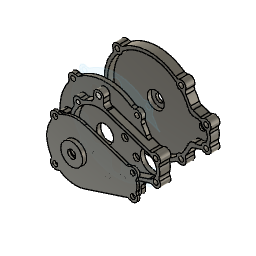
Gear Reduction Housing Assembly (v2~recovered) (Autodesk Fusion 360 design; units mm, degrees)
Autodesk Fusion 360 part; units mm, degrees
sketch "Layout Sketch" plane through (0, 0, 0) normal (0, 1, 0) x (1, 0, 0)
  circle A0 centre (0, 0) radius 48
  circle A1 centre (0, 0) radius 16
  circle A2 centre (58, 0) radius 10
  circle A3 centre (24.6564, -8.25) radius 10
  circle A4 centre (38.8667, 5.8237) radius 10
  line L0 (0, 0) -> (38.8667, 0) construction
  line L1 (38.8667, 0) -> (38.8667, 5.8237) construction
  line L2 (24.6564, -8.25) -> (24.6564, 0) construction
  circle A5 centre (38.8667, 5.8237) radius 14 construction
  circle A6 centre (24.6564, -8.25) radius 14 construction
  dimension "d12" = 96
  dimension "d13" = 32
  dimension "d14" = 20
  dimension "d15" = 20
  dimension "d16" = 20
  dimension "d55" = 4
  dimension "d56" = 8.25
  constraint coincident A0.centre A1.centre
  constraint concentric A0 A1
  constraint horizontal A0.centre A2.centre
  constraint tangent A0 A2
  constraint tangent A3 A4
  constraint tangent A1 A3
  constraint horizontal L0
  constraint coincident A4.centre L1.end
  constraint coincident A3.centre L2.start
  constraint coincident L0 L2.end
  constraint perpendicular L0 L2
  constraint perpendicular L0 L1
  constraint tangent A2 A4
  constraint concentric A4 A5
  constraint concentric A3 A6
  constraint equal A5 A6
  measures "d12" diameter of A0
  measures "d13" diameter of A1
  measures "d14" diameter of A2
  measures "d15" diameter of A3
  measures "d16" diameter of A4
  measures "d55" distance of A4 A5
  measures "d56" distance of A3.centre L2.end
sketch "Housing Layout Sketch" plane through (0, 0, 0) normal (0, 1, 0) x (1, 0, 0)
  circle A0 centre (0, 0) radius 56
  circle A1 centre (0, 0) radius 48 construction
  circle A2 centre (58, 0) radius 10 construction
  circle A3 centre (58, 0) radius 18
  circle A4 centre (39.598, 39.598) radius 6
  line L0 (0, 0) -> (0, 56) construction
  line L1 (0, 0) -> (39.598, 39.598) construction
  line L2 (0, 0) -> (-56, 0) construction
  circle A5 centre (-39.598, 39.598) radius 6
  circle A6 centre (-39.598, -39.598) radius 6
  circle A7 centre (39.598, -39.598) radius 6
  circle A8 centre (70.7279, -12.7279) radius 6
  line L3 (58, 0) -> (70.7279, -12.7279) construction
  circle A9 centre (70.7279, 12.7279) radius 6
  circle A10 centre (39.598, 39.598) radius 4
  circle A11 centre (-39.598, 39.598) radius 4
  circle A12 centre (-39.598, -39.598) radius 4
  circle A13 centre (39.598, -39.598) radius 4
  circle A14 centre (70.7279, -12.7279) radius 4
  circle A15 centre (70.7279, 12.7279) radius 4
  circle A16 centre (0, 0) radius 16 construction
  circle A17 centre (24.6564, -8.25) radius 10 construction
  circle A18 centre (38.8667, 5.8237) radius 10 construction
  circle A19 centre (0, 0) radius 36
  line L4 (11.1724, -34.2225) -> (63.5862, -17.1112)
  line L5 (11.1724, 34.2225) -> (63.5862, 17.1112)
  circle A20 centre (24.6564, -8.25) radius 4
  circle A21 centre (38.8667, 5.8237) radius 4
  circle A22 centre (58, 0) radius 4
  circle A23 centre (0, 0) radius 52
  circle A24 centre (0, 0) radius 5
  circle A25 centre (58, 0) radius 14
  dimension "Gear_Clearance_Drive" = 8
  dimension "d18" = 8
  dimension "d19" = 12
  dimension "d20" = 45
  dimension "d21" = 45
  dimension "d22" = 8
  dimension "d23" = 20
  dimension "d24" = 8
  dimension "d25" = 104
  dimension "d27" = 10
  dimension "d57" = 4
  constraint coincident A0.centre A1.centre
  constraint coincident A0 A4.centre
  constraint coincident A0 L0.end
  constraint vertical L0
  constraint coincident A4.centre L1.end
  constraint coincident A0 L2.end
  constraint perpendicular L0 L2
  constraint symmetric A4 L0 A5
  constraint coincident A0 A6.centre
  constraint symmetric L2 A5 A6
  constraint coincident A0 A7.centre
  constraint symmetric L0 A6 A7
  constraint coincident A3 A8.centre
  constraint coincident A2.centre A3.centre
  constraint coincident A8.centre L3.end
  constraint equal A4 A8
  constraint symmetric L2 A8 A9
  constraint concentric A4 A10
  constraint concentric A5 A11
  constraint concentric A6 A12
  constraint concentric A7 A13
  constraint concentric A8 A14
  constraint concentric A9 A15
  constraint equal A14 A15
  constraint equal A13 A14
  constraint equal A12 A13
  constraint equal A11 A12
  constraint equal A10 A11
  constraint concentric A16 A19
  constraint coincident A19 L4.start
  constraint coincident A3 L4.end
  constraint coincident A19 L5.start
  constraint coincident A3 L5.end
  constraint tangent A19 L4
  constraint tangent A3 L4
  constraint tangent A19 L5
  constraint tangent A3 L5
  constraint concentric A17 A20
  constraint concentric A18 A21
  constraint equal A21 A22
  constraint equal A20 A21
  constraint concentric A16 A23
  constraint concentric A23 A24
  constraint concentric A22 A25
  measures "Gear_Clearance_Drive" distance of A0 A1
  measures "d19" diameter of A4
  measures "d20" angle of L0 L1
  measures "d21" angle of L0 L3
  measures "d22" diameter of A10
  measures "d23" distance of A16 A19
  measures "d24" diameter of A22
  measures "d25" diameter of A23
  measures "d27" diameter of A24
  measures "d57" distance of A2 A25
ref_plane "WorkPlane1" through (0, 11, 0) normal (0, 1, 0) x (0, 0, 1)
ref_plane "WorkPlane2" through (0, -5, 0) normal (0, 1, 0) x (0, 0, 1)
ref_plane "WorkPlane3" through (0, -13, 0) normal (0, 1, 0) x (0, 0, 1)
extrude "Extrude1" add sketch "Housing Layout Sketch" along normal up to surface (11 mm away) contours A0 A22 | A0 A22 | A0 A22 A23 A25 | A0 A8 A9 A22 A25 | A0 A3 A23 A25 | A0 A3 A9 A25 | A0 A3 A8 A25 | A0 A3 A23 A25 | A0 A3 L5 A23 | A0 A3 L5 | A9 A25 | A3 A9 A15 A25 | A3 A21 A23 A25 | A23 A25 | A0 A3 L4 | A0 A3 L4 A23 | A3 A8 A14 A25 | A8 A25 | A0 A4 L5 A23 | A3 A19 L5 A21 A23 | A3 A9 A15 | A3 A9 A15 A25 | A3 A8 A9 A25 | A3 A15 | A0 A7 L4 A23 | A3 A19 L4 A21 A23 | A3 A8 A14 A25 | A3 A8 A14 | A3 A14 | A0 A4 A10 A23 | A0 A4 A10 | A4 A5 A6 A7 A19 L4 L5 A23 | A3 A21 | A3 A19 A21 | A3 A15 | A0 A7 A13 | A0 A7 A13 A23 | A3 A14 | A0 A10 | A0 A10 | A4 A23 | A19 A21 | A19 A21 | A0 A13 | A0 A13 | A7 A23 | A0 A4 A10 A23 | A0 A4 A5 A23 | A0 A7 A13 A23 | A0 A6 A7 A23 | A0 A5 A11 A23 | A5 A23 | A0 A5 A11 | A0 A6 A12 | A0 A6 A12 A23 | A6 A23 | A0 A5 A11 A23 | A0 A11 | A0 A11 | A0 A5 A6 A23 | A0 A12 | A0 A12 | A0 A6 A12 A23 | A20 | A24 makes body 1
extrude "Extrude2" add 1 faces at (5.6052, 0, -26.2324) along direction (0, -1, 0) up to surface (5 mm away) separate body on bodies 1 makes body 2
extrude "Extrude3" add sketch "Housing Layout Sketch" against normal up to surface (8 mm away) from surface at -5 separate body contours A0 A22 | A0 A22 | A0 A22 A23 A25 | A0 A8 A9 A22 A25 | A0 A3 A23 A25 | A0 A3 A9 A25 | A0 A3 A8 A25 | A0 A3 A23 A25 | A0 A3 L5 A23 | A0 A3 L5 | A9 A25 | A3 A9 A15 A25 | A3 A21 A23 A25 | A23 A25 | A0 A3 L4 | A0 A3 L4 A23 | A3 A8 A14 A25 | A8 A25 | A3 A19 L5 A21 A23 | A3 A9 A15 | A3 A9 A15 A25 | A3 A8 A9 A25 | A3 A15 | A3 A19 L4 A21 A23 | A3 A8 A14 A25 | A3 A8 A14 | A3 A14 | A3 A21 | A3 A19 A21 | A3 A15 | A3 A14 | A19 A21 | A19 A21 | A20 | A24 makes body 3
extrude "Extrude4" add 1 faces at (-6.1142, -13, -2.1538) along direction (0, -1, 0) blind 3 separate body on bodies 3 makes body 4
combine "Combine1" operation add target body 2 tool bodies 3
sketch "Front Cover Cut" plane through (0, -13, 0) normal (0, -1, 0) x (1, 0, 0)
  arc A0 (65.8375, 16.2041) -> (63.5862, 17.1112) centre (58, 0) ccw
  line L0 (63.5862, 17.1112) -> (11.1724, 34.2225)
  arc A1 (11.1724, 34.2225) -> (11.1724, -34.2225) centre (0, 0) ccw
  line L1 (11.1724, -34.2225) -> (63.5862, -17.1112)
  arc A2 (63.5862, -17.1112) -> (65.8375, -16.2041) centre (58, 0) ccw
  arc A3 (65.8375, -16.2041) -> (74.2041, -7.8375) centre (70.7279, -12.7279) ccw
  arc A4 (74.2041, -7.8375) -> (74.2041, 7.8375) centre (58, 0) ccw
  arc A5 (74.2041, 7.8375) -> (65.8375, 16.2041) centre (70.7279, 12.7279) ccw
  line L2 (11.1724, 34.2225) -> (63.5862, 17.1112)
  circle A6 centre (0, 0) radius 36 construction
  circle A7 centre (58, 0) radius 18 construction
  line L3 (11.1724, -34.2225) -> (63.5862, -17.1112)
  arc A8 (11.1724, 34.2225) -> (11.1724, -34.2225) centre (0, 0) ccw
  arc A9 (63.5862, -17.1112) -> (63.5862, 17.1112) centre (58, 0) ccw
  arc A10 (62.3448, -13.3087) -> (62.3448, 13.3087) centre (58, 0) ccw
  line L4 (62.3448, 13.3087) -> (9.931, 30.42)
  arc A11 (9.931, 30.42) -> (9.931, -30.42) centre (0, 0) ccw
  line L5 (9.931, -30.42) -> (62.3448, -13.3087)
  dimension "d44" = -4
  constraint coincident A1.end L1.start
  constraint coincident L0.end A1.start
  constraint tangent L0 A8
  constraint coincident A0.end L0.start
  constraint coincident L1.end A2.start
  constraint tangent L3 A9
extrude "Extrude5" cut sketch "Front Cover Cut" against normal up to surface (8 mm away) contours A10 L4 A11 L5 bodies 2
sketch "Main Bearing OD" plane through (0, 0, 0) normal (0, 1, 0) x (1, 0, 0)
  circle A0 centre (0, 0) radius 10.5
  dimension "d47" = 21
  constraint coincident A0.centre origin
  measures "d47" diameter of A0
extrude "Extrude6" cut sketch "Main Bearing OD" along normal through all and the other way through all bodies 1 2 4
sketch "Cover Bearing" plane through (0, 0, 0) normal (1, 0, 0) x (0, 1, 0)
  line L0 (-13, -10.5) -> (-16, -10.5)
  line L1 (-16, 10.5) -> (-13, 10.5)
  line L2 (-16, 10.5) -> (-18, 10.5)
  line L3 (-18, 10.5) -> (-18, 5)
  line L4 (-18, 5) -> (-21, 5)
  line L5 (-21, 5) -> (-21, 13.5)
  line L6 (-21, 13.5) -> (-16, 13.5)
  line L7 (-16, 13.5) -> (-16, 10.5)
  line L8 (0, 0) -> (-21.9581, 0) construction
  line L9 (11, -10.5) -> (0, -10.5)
  line L10 (0, 10.5) -> (11, 10.5)
  line L11 (11, 10.5) -> (13, 10.5)
  line L12 (13, 10.5) -> (13, 5)
  line L13 (13, 5) -> (16, 5)
  line L14 (16, 5) -> (16, 13.5)
  line L15 (16, 13.5) -> (11, 13.5)
  line L16 (11, 13.5) -> (11, 10.5)
  dimension "d49" = 5
  dimension "d50" = 3
  dimension "d51" = 3
  dimension "d52" = 10
  constraint coincident L1.start L2.start
  constraint parallel L1 L2
  constraint perpendicular L2 L3
  constraint perpendicular L3 L4
  constraint perpendicular L2 L5
  constraint perpendicular L5 L6
  constraint perpendicular L2 L7
  constraint coincident L8.start origin
  constraint parallel L6 L8
  constraint coincident L10.end L11.start
  constraint parallel L10 L11
  constraint perpendicular L11 L12
  constraint perpendicular L12 L13
  constraint perpendicular L13 L14
  constraint perpendicular L14 L15
  constraint collinear L6 L15
  constraint equal L6 L15
  constraint equal L4 L13
  constraint equal L2 L11
  constraint collinear L4 L13
  measures "d49" distance of L1.end L3
  measures "d50" distance of L3.end L4.end
  measures "d51" distance of L6.end L1.start
revolve "Revolve1" add sketch "Cover Bearing" angle 360 about axis through (0, 0, 0) along (0, -1, 0) contours L2 L3 L4 L5 L6 L7 bodies 4
revolve "Revolve2" add sketch "Cover Bearing" angle 360 about axis through (0, 0, 0) along (0, -1, 0) contours L11 L12 L13 L14 L15 L16 bodies 1
extrude "Extrude7" cut sketch "Housing Layout Sketch" along normal blind 8 contours A0 A22 | A0 A22 | A0 A22 A23 A25 | A0 A8 A9 A22 A25 | A3 A21 A23 A25 | A23 A25 | A3 A19 L5 A21 A23 | A3 A19 L4 A21 A23 | A4 A5 A6 A7 A19 L4 L5 A23 | A3 A21 | A3 A19 A21 | A19 A21 | A19 A21 | A20 bodies 1
fillet "Fillet1" radius 8 2 edges at (50.6207, 4, 11.8973) (50.6207, 4, -11.8973) on bodies 1
extrude "Extrude8" cut sketch "Housing Layout Sketch" along normal blind 2 from surface at 8 contours A0 A22 | A0 A22 bodies 1
extrude "Extrude9" cut sketch "Housing Layout Sketch" against normal through all contours A0 A22 | A0 A22 | A0 A22 A23 A25 | A0 A8 A9 A22 A25 | A9 A25 | A23 A25 | A8 A25 bodies 2
extrude "Extrude10" cut sketch "Housing Layout Sketch" along normal blind 3 from surface at -5 contours A3 A21 | A3 A19 A21 | A19 A21 | A20 picked at (35.3672, 5.2993) bodies 2
extrude "Extrude11" cut sketch "Housing Layout Sketch" against normal blind 2 from surface at -13 contours A0 A22 | A0 A22 | A3 A21 | A3 A19 A21 | A19 A21 | A20 picked at (35.3672, 5.2993) bodies 4
fillet "Fillet2" radius 5 32 edges at (43.6072, 5.5, 35.1341) (35.1341, 5.5, 43.6072) (51.9496, 5.5, 20.9102) (65.8375, 5.5, 16.2041) (74.2041, 5.5, 7.8375) (74.2041, 5.5, -7.8375) (65.8375, 5.5, -16.2041) (51.9496, 5.5, -20.9102) (43.6072, 5.5, -35.1341) (35.1341, 5.5, -43.6072) (-35.1341, 5.5, -43.6072) (-43.6072, 5.5, -35.1341) (-43.6072, 5.5, 35.1341) (-35.1341, 5.5, 43.6072) (43.6072, -2.5, 35.1341) (35.1341, -2.5, 43.6072) (51.9496, -2.5, 20.9102) (65.8375, -6.5, 16.2041) (74.2041, -6.5, 7.8375) (74.2041, -6.5, -7.8375) (65.8375, -6.5, -16.2041) (51.9496, -2.5, -20.9102) (43.6072, -2.5, -35.1341) (35.1341, -2.5, -43.6072) (-35.1341, -2.5, -43.6072) (-43.6072, -2.5, -35.1341) (-43.6072, -2.5, 35.1341) (-35.1341, -2.5, 43.6072) (65.8375, -14.5, 16.2041) (74.2041, -14.5, 7.8375) (74.2041, -14.5, -7.8375) (65.8375, -14.5, -16.2041) on bodies 1 2 4
sketch "Main Hole Locations" plane through (0, -5, 0) normal (0, -1, 0) x (1, 0, 0)
  line L0 (11.1724, 34.2225) -> (54.1086, 20.2053)
  arc A0 (51.098, 22.9127) -> (54.1086, 20.2053) centre (55.6604, 24.9584) ccw
  arc A1 (51.098, 22.9127) -> (45.6564, 32.4267) centre (0, 0) ccw
  arc A2 (45.1261, 37.2656) -> (45.6564, 32.4267) centre (49.7329, 35.322) ccw
  arc A3 (45.1261, 37.2656) -> (37.2656, 45.1261) centre (39.598, 39.598) ccw
  arc A4 (32.4267, 45.6564) -> (37.2656, 45.1261) centre (35.322, 49.7329) ccw
  arc A5 (32.4267, 45.6564) -> (-32.4267, 45.6564) centre (0, 0) ccw
  arc A6 (-37.2656, 45.1261) -> (-32.4267, 45.6564) centre (-35.322, 49.7329) ccw
  arc A7 (-37.2656, 45.1261) -> (-45.1261, 37.2656) centre (-39.598, 39.598) ccw
  arc A8 (-45.6564, 32.4267) -> (-45.1261, 37.2656) centre (-49.7329, 35.322) ccw
  arc A9 (-45.6564, 32.4267) -> (-45.6564, -32.4267) centre (0, 0) ccw
  arc A10 (-45.1261, -37.2656) -> (-45.6564, -32.4267) centre (-49.7329, -35.322) ccw
  arc A11 (-45.1261, -37.2656) -> (-37.2656, -45.1261) centre (-39.598, -39.598) ccw
  arc A12 (-32.4267, -45.6564) -> (-37.2656, -45.1261) centre (-35.322, -49.7329) ccw
  arc A13 (-32.4267, -45.6564) -> (32.4267, -45.6564) centre (0, 0) ccw
  arc A14 (37.2656, -45.1261) -> (32.4267, -45.6564) centre (35.322, -49.7329) ccw
  arc A15 (37.2656, -45.1261) -> (45.1261, -37.2656) centre (39.598, -39.598) ccw
  arc A16 (45.6564, -32.4267) -> (45.1261, -37.2656) centre (49.7329, -35.322) ccw
  arc A17 (45.6564, -32.4267) -> (51.098, -22.9127) centre (0, 0) ccw
  arc A18 (54.1086, -20.2053) -> (51.098, -22.9127) centre (55.6604, -24.9584) ccw
  line L1 (54.1086, -20.2053) -> (11.1724, -34.2225)
  arc A19 (11.1724, 34.2225) -> (11.1724, -34.2225) centre (0, 0) ccw
  point P0 (-39.598, 39.598)
  point P1 (39.598, 39.598)
  point P2 (39.598, -39.598)
  point P3 (-39.598, -39.598)
  constraint coincident P0 A7.centre
  constraint coincident P1 A3.centre
  constraint coincident P2 A15.centre
  constraint coincident P3 A11.centre
hole "Hole1" at (39.598, -5, 39.598) at (-39.598, -5, 39.598) at (-39.598, -5, -39.598) at (39.598, -5, -39.598) direction (0, 1, 0) diameter 6 end through all bodies 1 2
sketch "Secondary Hole Locations" plane through (0, -16, 0) normal (0, -1, 0) x (1, 0, 0)
  circle A0 centre (0, 0) radius 13.5
  arc A1 (63.2283, 17.2281) -> (67.4836, 17.7752) centre (64.7801, 21.9812) ccw
  line L0 (63.2283, 17.2281) -> (11.1724, 34.2225)
  arc A2 (11.1724, 34.2225) -> (11.1724, -34.2225) centre (0, 0) ccw
  line L1 (11.1724, -34.2225) -> (63.2283, -17.2281)
  arc A3 (67.4836, -17.7752) -> (63.2283, -17.2281) centre (64.7801, -21.9812) ccw
  arc A4 (67.4836, -17.7752) -> (75.774, -9.4818) centre (70.7279, -12.7279) ccw
  arc A5 (75.201, -5.3035) -> (75.774, -9.4818) centre (79.979, -6.7767) ccw
  arc A6 (75.201, -5.3035) -> (75.201, 5.3035) centre (58, 0) ccw
  arc A7 (75.774, 9.4818) -> (75.201, 5.3035) centre (79.979, 6.7767) ccw
  arc A8 (75.774, 9.4818) -> (67.4836, 17.7752) centre (70.7279, 12.7279) ccw
  point P0 (70.7279, 12.7279)
  point P1 (70.7279, -12.7279)
  constraint coincident P0 A8.centre
  constraint coincident P1 A4.centre
hole "Hole2" at (70.7279, -16, 12.7279) at (70.7279, -16, -12.7279) direction (0, 1, 0) diameter 6 end through all bodies 1 2 4
sketch "Front Cover Mounting Holes" plane through (0, -16, 0) normal (0, -1, 0) x (1, 0, 0)
  circle A0 centre (70.7279, 12.7279) radius 3
  circle A1 centre (70.7279, -12.7279) radius 3
  circle A2 centre (0, 0) radius 13.5
  arc A3 (63.2283, 17.2281) -> (67.4836, 17.7752) centre (64.7801, 21.9812) ccw
  line L0 (63.2283, 17.2281) -> (11.1724, 34.2225)
  arc A4 (11.1724, 34.2225) -> (11.1724, -34.2225) centre (0, 0) ccw
  line L1 (11.1724, -34.2225) -> (63.2283, -17.2281)
  arc A5 (67.4836, -17.7752) -> (63.2283, -17.2281) centre (64.7801, -21.9812) ccw
  arc A6 (67.4836, -17.7752) -> (75.774, -9.4818) centre (70.7279, -12.7279) ccw
  arc A7 (75.201, -5.3035) -> (75.774, -9.4818) centre (79.979, -6.7767) ccw
  arc A8 (75.201, -5.3035) -> (75.201, 5.3035) centre (58, 0) ccw
  arc A9 (75.774, 9.4818) -> (75.201, 5.3035) centre (79.979, 6.7767) ccw
  arc A10 (75.774, 9.4818) -> (67.4836, 17.7752) centre (70.7279, 12.7279) ccw
  line L2 (0, 0) -> (-36, 0) construction
  line L3 (0, 0) -> (-25.4558, 25.4558) construction
  circle A11 centre (-25.4558, 25.4558) radius 6
  circle A12 centre (-25.4558, -25.4558) radius 6
  dimension "d81" = 45
  dimension "d82" = 12
  constraint coincident A2.centre A4.centre
  constraint midpoint A4 L2.end
  constraint coincident A4 L3.end
  constraint coincident L3.end A11.centre
  constraint symmetric L2 A11 A12
  measures "d81" angle of L2 L3
  measures "d82" diameter of A11
extrude "Extrude12" add sketch "Front Cover Mounting Holes" against normal up to surface (3 mm away) contours A4 A11 | A4 A12 picked at (-26.9418, 26.7385) picked at (-26.9418, -26.7385) bodies 4
extrude "Extrude13" add sketch "Front Cover Mounting Holes" against normal up to surface (8 mm away) from surface at -3 contours A4 A11 | A4 A12 picked at (-26.9418, 26.7385) picked at (-26.9418, -26.7385) bodies 2
hole "Hole3" at (-25.4558, -16, 25.4558) at (-25.4558, -16, -25.4558) direction (0, 1, 0) diameter 6 depth 27 tip angle 180 bodies 4
hole "Hole4" at (-25.4558, -16, 25.4558) at (-25.4558, -16, -25.4558) direction (0, 1, 0) diameter 5.035 depth 27 tip angle 180 bodies 2
thread "Thread1" "ISO Metric profile 6.0 M6x1 6H" thread offset 0 thread depth 10
sketch "Housing Mount" plane through (0, -5, 0) normal (0, -1, 0) x (1, 0, 0)
  arc A0 (-29.3302, -20.8744) -> (-20.8744, -29.3302) centre (-25.4558, -25.4558) ccw
  arc A1 (-29.3302, 20.8744) -> (-29.3302, -20.8744) centre (0, 0) ccw
  arc A2 (-20.8744, 29.3302) -> (-29.3302, 20.8744) centre (-25.4558, 25.4558) ccw
  arc A3 (11.1724, 34.2225) -> (-20.8744, 29.3302) centre (0, 0) ccw
  line L0 (11.1724, 34.2225) -> (54.1086, 20.2053)
  arc A4 (51.098, 22.9127) -> (54.1086, 20.2053) centre (55.6604, 24.9584) ccw
  arc A5 (51.098, 22.9127) -> (45.6564, 32.4267) centre (0, 0) ccw
  arc A6 (45.1261, 37.2656) -> (45.6564, 32.4267) centre (49.7329, 35.322) ccw
  arc A7 (45.1261, 37.2656) -> (37.2656, 45.1261) centre (39.598, 39.598) ccw
  arc A8 (32.4267, 45.6564) -> (37.2656, 45.1261) centre (35.322, 49.7329) ccw
  arc A9 (32.4267, 45.6564) -> (-32.4267, 45.6564) centre (0, 0) ccw
  arc A10 (-37.2656, 45.1261) -> (-32.4267, 45.6564) centre (-35.322, 49.7329) ccw
  arc A11 (-37.2656, 45.1261) -> (-45.1261, 37.2656) centre (-39.598, 39.598) ccw
  arc A12 (-45.6564, 32.4267) -> (-45.1261, 37.2656) centre (-49.7329, 35.322) ccw
  arc A13 (-45.6564, 32.4267) -> (-45.6564, -32.4267) centre (0, 0) ccw
  arc A14 (-45.1261, -37.2656) -> (-45.6564, -32.4267) centre (-49.7329, -35.322) ccw
  arc A15 (-45.1261, -37.2656) -> (-37.2656, -45.1261) centre (-39.598, -39.598) ccw
  arc A16 (-32.4267, -45.6564) -> (-37.2656, -45.1261) centre (-35.322, -49.7329) ccw
  arc A17 (-32.4267, -45.6564) -> (32.4267, -45.6564) centre (0, 0) ccw
  arc A18 (37.2656, -45.1261) -> (32.4267, -45.6564) centre (35.322, -49.7329) ccw
  arc A19 (37.2656, -45.1261) -> (45.1261, -37.2656) centre (39.598, -39.598) ccw
  arc A20 (45.6564, -32.4267) -> (45.1261, -37.2656) centre (49.7329, -35.322) ccw
  arc A21 (45.6564, -32.4267) -> (51.098, -22.9127) centre (0, 0) ccw
  arc A22 (54.1086, -20.2053) -> (51.098, -22.9127) centre (55.6604, -24.9584) ccw
  line L1 (54.1086, -20.2053) -> (11.1724, -34.2225)
  arc A23 (-20.8744, -29.3302) -> (11.1724, -34.2225) centre (0, 0) ccw
  circle A24 centre (39.598, -39.598) radius 3
  circle A25 centre (-39.598, 39.598) radius 3
  circle A26 centre (39.598, 39.598) radius 3
  circle A27 centre (-39.598, -39.598) radius 3
  circle A28 centre (0, 45) radius 6
  dimension "d94" = 45
  dimension "d95" = 12
  constraint vertical A1.centre A28.centre
  measures "d94" distance of A1.centre A28.centre
  measures "d95" diameter of A28
extrude "Extrude14" add sketch "Housing Mount" along normal up to surface (8 mm away) contours A28 bodies 2
hole "Hole5" at (0, -13, 45) direction (0, 1, 0) diameter 6.78 depth 27 tip angle 180 bodies 2
thread "Thread2" "ISO Metric profile 8.0 M8x1.25 6H" thread offset 0 thread depth 10
pattern_circular "C-Pattern1" count 3 over 180 about axis through (0, -5, 0) along (0, -1, 0) of "Extrude14", "Hole5"
sketch "Housing Mount Support" plane through (0, -13, 0) normal (0, -1, 0) x (1, 0, 0)
  circle A0 centre (-25.4558, 25.4558) radius 2.5175
  circle A1 centre (-25.4558, -25.4558) radius 2.5175
  circle A2 centre (70.7279, 12.7279) radius 3
  circle A3 centre (70.7279, -12.7279) radius 3
  line L0 (62.3448, -13.3087) -> (9.931, -30.42)
  arc A4 (9.931, 30.42) -> (9.931, -30.42) centre (0, 0) ccw
  line L1 (9.931, 30.42) -> (62.3448, 13.3087)
  arc A5 (62.3448, -13.3087) -> (62.3448, 13.3087) centre (58, 0) ccw
  line L2 (63.2283, 17.2281) -> (11.1724, 34.2225)
  arc A6 (11.1724, 34.2225) -> (-20.8744, 29.3302) centre (0, 0) ccw
  arc A7 (-20.8744, 29.3302) -> (-29.3302, 20.8744) centre (-25.4558, 25.4558) ccw
  arc A8 (-29.3302, 20.8744) -> (-29.3302, -20.8744) centre (0, 0) ccw
  arc A9 (-29.3302, -20.8744) -> (-20.8744, -29.3302) centre (-25.4558, -25.4558) ccw
  arc A10 (-20.8744, -29.3302) -> (11.1724, -34.2225) centre (0, 0) ccw
  line L3 (11.1724, -34.2225) -> (63.2283, -17.2281)
  arc A11 (67.4836, -17.7752) -> (63.2283, -17.2281) centre (64.7801, -21.9812) ccw
  arc A12 (67.4836, -17.7752) -> (75.774, -9.4818) centre (70.7279, -12.7279) ccw
  arc A13 (75.201, -5.3035) -> (75.774, -9.4818) centre (79.979, -6.7767) ccw
  arc A14 (75.201, -5.3035) -> (75.201, 5.3035) centre (58, 0) ccw
  arc A15 (75.774, 9.4818) -> (75.201, 5.3035) centre (79.979, 6.7767) ccw
  arc A16 (75.774, 9.4818) -> (67.4836, 17.7752) centre (70.7279, 12.7279) ccw
  arc A17 (63.2283, 17.2281) -> (67.4836, 17.7752) centre (64.7801, 21.9812) ccw
  circle A18 centre (0, 45) radius 6
  circle A19 centre (-45, 0) radius 6
  circle A20 centre (0, -45) radius 6
  line L4 (-6, 45) -> (-6, 35.4965)
  line L5 (6, 45) -> (6, 35.4965)
  constraint coincident A18 L4.start
  constraint coincident A6 L4.end
  constraint vertical L4
  constraint coincident A18 L5.start
  constraint coincident A6 L5.end
  constraint parallel L4 L5
  constraint tangent A18 L5
  constraint tangent A18 L4
extrude "Extrude15" add sketch "Housing Mount Support" against normal up to surface (8 mm away) contours A6 A18 L4 L5 bodies 2
pattern_circular "C-Pattern2" count 3 over 180 about axis through (0, -5, 0) along (0, -1, 0) of "Extrude15"
fillet "Fillet4" radius 5 14 edges at (-20.8744, -9, -29.3302) (-6, -9, -35.4965) (6, -9, -35.4965) (-29.3302, -9, -20.8744) (-35.4965, -9, -6) (-35.4965, -9, 6) (-29.3302, -9, 20.8744) (-20.8744, -9, 29.3302) (-6, -9, 35.4965) (6, -9, 35.4965) (-20.8744, -14.5, -29.3302) (-29.3302, -14.5, -20.8744) (-29.3302, -14.5, 20.8744) (-20.8744, -14.5, 29.3302) on bodies 2 4
sketch "External Mount Sketch" plane through (0, -13, 0) normal (0, -1, 0) x (1, 0, 0)
  circle A0 centre (-45, 0) radius 3.3898
  circle A1 centre (0, 45) radius 3.3898
  circle A2 centre (-25.4558, 25.4558) radius 2.5175
  circle A3 centre (-25.4558, -25.4558) radius 2.5175
  circle A4 centre (70.7279, 12.7279) radius 3
  circle A5 centre (70.7279, -12.7279) radius 3
  line L0 (62.3448, -13.3087) -> (9.931, -30.42)
  arc A6 (9.931, 30.42) -> (9.931, -30.42) centre (0, 0) ccw
  line L1 (9.931, 30.42) -> (62.3448, 13.3087)
  arc A7 (62.3448, -13.3087) -> (62.3448, 13.3087) centre (58, 0) ccw
  circle A8 centre (0, -45) radius 3.3898
  arc A9 (-6, -45) -> (6, -45) centre (0, -45) ccw
  line L2 (6, -45) -> (6, -39.4968)
  arc A10 (9.6585, -34.6801) -> (6, -39.4968) centre (11, -39.4968) ccw
  arc A11 (9.6585, -34.6801) -> (11.1724, -34.2225) centre (0, 0) ccw
  line L3 (11.1724, -34.2225) -> (63.2283, -17.2281)
  arc A12 (67.4836, -17.7752) -> (63.2283, -17.2281) centre (64.7801, -21.9812) ccw
  arc A13 (67.4836, -17.7752) -> (75.774, -9.4818) centre (70.7279, -12.7279) ccw
  arc A14 (75.201, -5.3035) -> (75.774, -9.4818) centre (79.979, -6.7767) ccw
  arc A15 (75.201, -5.3035) -> (75.201, 5.3035) centre (58, 0) ccw
  arc A16 (75.774, 9.4818) -> (75.201, 5.3035) centre (79.979, 6.7767) ccw
  arc A17 (75.774, 9.4818) -> (67.4836, 17.7752) centre (70.7279, 12.7279) ccw
  arc A18 (63.2283, 17.2281) -> (67.4836, 17.7752) centre (64.7801, 21.9812) ccw
  line L4 (63.2283, 17.2281) -> (11.1724, 34.2225)
  arc A19 (11.1724, 34.2225) -> (9.6585, 34.6801) centre (0, 0) ccw
  arc A20 (6, 39.4968) -> (9.6585, 34.6801) centre (11, 39.4968) ccw
  line L5 (6, 39.4968) -> (6, 45)
  arc A21 (6, 45) -> (-6, 45) centre (0, 45) ccw
  line L6 (-6, 45) -> (-6, 39.4968)
  arc A22 (-9.6585, 34.6801) -> (-6, 39.4968) centre (-11, 39.4968) ccw
  arc A23 (-9.6585, 34.6801) -> (-18.189, 31.067) centre (0, 0) ccw
  arc A24 (-22.8701, 30.8701) -> (-18.189, 31.067) centre (-20.7152, 35.3819) ccw
  arc A25 (-22.8701, 30.8701) -> (-30.8701, 22.8701) centre (-25.4558, 25.4558) ccw
  arc A26 (-31.067, 18.189) -> (-30.8701, 22.8701) centre (-35.3819, 20.7152) ccw
  arc A27 (-31.067, 18.189) -> (-34.6801, 9.6585) centre (0, 0) ccw
  arc A28 (-39.4968, 6) -> (-34.6801, 9.6585) centre (-39.4968, 11) ccw
  line L7 (-39.4968, 6) -> (-45, 6)
  arc A29 (-45, 6) -> (-45, -6) centre (-45, 0) ccw
  line L8 (-45, -6) -> (-39.4968, -6)
  arc A30 (-34.6801, -9.6585) -> (-39.4968, -6) centre (-39.4968, -11) ccw
  arc A31 (-34.6801, -9.6585) -> (-31.067, -18.189) centre (0, 0) ccw
  arc A32 (-30.8701, -22.8701) -> (-31.067, -18.189) centre (-35.3819, -20.7152) ccw
  arc A33 (-30.8701, -22.8701) -> (-22.8701, -30.8701) centre (-25.4558, -25.4558) ccw
  arc A34 (-18.189, -31.067) -> (-22.8701, -30.8701) centre (-20.7152, -35.3819) ccw
  arc A35 (-18.189, -31.067) -> (-9.6585, -34.6801) centre (0, 0) ccw
  arc A36 (-6, -39.4968) -> (-9.6585, -34.6801) centre (-11, -39.4968) ccw
  line L9 (-6, -39.4968) -> (-6, -45)
  circle A37 centre (0, 45) radius 6
  circle A38 centre (-45, 0) radius 6
  circle A39 centre (0, -45) radius 6
  circle A40 centre (0, 45) radius 9
  circle A41 centre (0, -45) radius 9
  arc A42 (0, 54) -> (0, -54) centre (0, 0) ccw
  arc A43 (-8.535, 42.1444) -> (-8.535, -42.1444) centre (0, 0) ccw
  circle A44 centre (-45, 0) radius 9
  dimension "d108" = 108
  dimension "d109" = 12
  dimension "d110" = 12
  dimension "d111" = 12
  dimension "d112" = 43
  constraint concentric A6 A42
  constraint concentric A1 A37
  constraint concentric A0 A38
  constraint concentric A8 A39
  constraint concentric A1 A40
  constraint tangent A40 A42
  constraint concentric A39 A41
  constraint tangent A41 A42
  constraint coincident A40 A42.start
  constraint coincident A41 A42.end
  constraint coincident A40 A43.start
  constraint coincident A41 A43.end
  constraint concentric A42 A43
  constraint concentric A0 A44
  constraint tangent A42 A44
  measures "d108" diameter of A42
  measures "d109" diameter of A37
  measures "d110" diameter of A38
  measures "d111" diameter of A39
  measures "d112" radius of A43
extrude "Extrude1'" add sketch "External Mount Sketch" along normal blind 10 separate body contours A0 A38 A43 | A0 A29 A38 A43 | A28 L7 L8 A30 A38 A43 A44 | L7 A38 A43 | L8 A38 A43 | L7 A29 L8 A38 A43 A44 | A28 L7 A43 A44 | L8 A30 A43 A44 | A40 A42 A43 A44 | A41 A42 A43 A44 | A20 L5 A21 L6 A22 A37 A40 | A9 L2 A10 A36 L9 A39 A41 | A20 L5 L6 A22 A37 A40 | L2 A10 A36 L9 A39 A41 | A21 A37 | A9 A39 makes body 5 in component "gear house mount"
copy_body "Body->Comp1" bodies 1 removing the originals makes body 6 in component "Back Housing"
copy_body "Body->Comp2" bodies 2 removing the originals makes body 7 in component "Front Housing"
copy_body "Body->Comp3" bodies 4 removing the originals makes body 8 in component "Front Cover"
sketch "Sketch12" plane through (28.9691, -5, 10.3013) normal (0, -1, 0) x (1, 0, 0)
  arc A0 (-22.9691, 29.1955) -> (-19.3106, 24.3788) centre (-17.9691, 29.1955) ccw
  arc A1 (-17.7967, 23.9211) -> (-19.3106, 24.3788) centre (-28.9691, -10.3013) ccw
  line L0 (-17.7967, 23.9211) -> (25.1395, 9.904)
  arc A2 (22.1289, 12.6113) -> (25.1395, 9.904) centre (26.6913, 14.6571) ccw
  arc A3 (22.1289, 12.6113) -> (16.6873, 22.1254) centre (-28.9691, -10.3013) ccw
  arc A4 (16.157, 26.9643) -> (16.6873, 22.1254) centre (20.7638, 25.0206) ccw
  arc A5 (16.157, 26.9643) -> (8.2965, 34.8248) centre (10.6289, 29.2966) ccw
  arc A6 (3.4576, 35.3551) -> (8.2965, 34.8248) centre (6.3529, 39.4315) ccw
  arc A7 (3.4576, 35.3551) -> (-61.3958, 35.3551) centre (-28.9691, -10.3013) ccw
  arc A8 (-66.2347, 34.8248) -> (-61.3958, 35.3551) centre (-64.2911, 39.4315) ccw
  arc A9 (-66.2347, 34.8248) -> (-74.0952, 26.9643) centre (-68.5671, 29.2966) ccw
  arc A10 (-74.6255, 22.1254) -> (-74.0952, 26.9643) centre (-78.702, 25.0206) ccw
  arc A11 (-74.6255, 22.1254) -> (-74.6255, -42.7281) centre (-28.9691, -10.3013) ccw
  arc A12 (-74.0952, -47.567) -> (-74.6255, -42.7281) centre (-78.702, -45.6233) ccw
  arc A13 (-74.0952, -47.567) -> (-66.2347, -55.4274) centre (-68.5671, -49.8993) ccw
  arc A14 (-61.3958, -55.9577) -> (-66.2347, -55.4274) centre (-64.2911, -60.0342) ccw
  arc A15 (-61.3958, -55.9577) -> (3.4576, -55.9577) centre (-28.9691, -10.3013) ccw
  arc A16 (8.2965, -55.4274) -> (3.4576, -55.9577) centre (6.3529, -60.0342) ccw
  arc A17 (8.2965, -55.4274) -> (16.157, -47.567) centre (10.6289, -49.8993) ccw
  arc A18 (16.6873, -42.7281) -> (16.157, -47.567) centre (20.7638, -45.6233) ccw
  arc A19 (16.6873, -42.7281) -> (22.1289, -33.214) centre (-28.9691, -10.3013) ccw
  arc A20 (25.1395, -30.5067) -> (22.1289, -33.214) centre (26.6913, -35.2598) ccw
  line L1 (25.1395, -30.5067) -> (-17.7967, -44.5238)
  arc A21 (-19.3106, -44.9815) -> (-17.7967, -44.5238) centre (-28.9691, -10.3013) ccw
  arc A22 (-19.3106, -44.9815) -> (-22.9691, -49.7982) centre (-17.9691, -49.7982) ccw
  line L2 (-22.9691, -49.7982) -> (-22.9691, -55.3013)
  arc A23 (-34.9691, -55.3013) -> (-22.9691, -55.3013) centre (-28.9691, -55.3013) ccw
  line L3 (-34.9691, -55.3013) -> (-34.9691, -49.7982)
  arc A24 (-34.9691, -49.7982) -> (-38.6276, -44.9815) centre (-39.9691, -49.7982) ccw
  arc A25 (-47.1581, -41.3684) -> (-38.6276, -44.9815) centre (-28.9691, -10.3013) ccw
  arc A26 (-47.1581, -41.3684) -> (-51.8392, -41.1714) centre (-49.6843, -45.6832) ccw
  arc A27 (-59.8392, -33.1714) -> (-51.8392, -41.1714) centre (-54.4249, -35.7572) ccw
  arc A28 (-59.8392, -33.1714) -> (-60.0361, -28.4903) centre (-64.351, -31.0166) ccw
  arc A29 (-63.6493, -19.9599) -> (-60.0361, -28.4903) centre (-28.9691, -10.3013) ccw
  arc A30 (-63.6493, -19.9599) -> (-68.4659, -16.3013) centre (-68.4659, -21.3013) ccw
  line L4 (-68.4659, -16.3013) -> (-73.9691, -16.3013)
  arc A31 (-73.9691, -4.3013) -> (-73.9691, -16.3013) centre (-73.9691, -10.3013) ccw
  line L5 (-73.9691, -4.3013) -> (-68.4659, -4.3013)
  arc A32 (-68.4659, -4.3013) -> (-63.6493, -0.6428) centre (-68.4659, 0.6987) ccw
  arc A33 (-60.0361, 7.8876) -> (-63.6493, -0.6428) centre (-28.9691, -10.3013) ccw
  arc A34 (-60.0361, 7.8876) -> (-59.8392, 12.5687) centre (-64.351, 10.4139) ccw
  arc A35 (-51.8392, 20.5687) -> (-59.8392, 12.5687) centre (-54.4249, 15.1545) ccw
  arc A36 (-51.8392, 20.5687) -> (-47.1581, 20.7657) centre (-49.6843, 25.0806) ccw
  arc A37 (-38.6276, 24.3788) -> (-47.1581, 20.7657) centre (-28.9691, -10.3013) ccw
  arc A38 (-38.6276, 24.3788) -> (-34.9691, 29.1955) centre (-39.9691, 29.1955) ccw
  line L6 (-34.9691, 29.1955) -> (-34.9691, 34.6987)
  arc A39 (-22.9691, 34.6987) -> (-34.9691, 34.6987) centre (-28.9691, 34.6987) ccw
  line L7 (-22.9691, 34.6987) -> (-22.9691, 29.1955)
  circle A40 centre (10.6289, -49.8993) radius 3
  circle A41 centre (-68.5671, 29.2966) radius 3
  circle A42 centre (10.6289, 29.2966) radius 3
  circle A43 centre (-68.5671, -49.8993) radius 3
component "gear house mount" placed x (1, 0, 0) y (0, 1, 0) z (0, 0, 1) at (0, 0, 0)
component "gear housing" placed x (1, 0, 0) y (0, 1, 0) z (0, 0, 1) at (0, 0, 0)
component "Back Housing" placed x (1, 0, 0) y (0, 1, 0) z (0, 0, 1) at (0, 0, 0) in component "gear housing"
component "Front Housing" placed x (1, 0, 0) y (0, 1, 0) z (0, 0, 1) at (0, 0, 0) in component "gear housing"
component "Front Cover" placed x (1, 0, 0) y (0, 1, 0) z (0, 0, 1) at (0, 0, 0) in component "gear housing"
equation "Drive_Gear_Teeth = 48"
equation "Driven_Gear_Teeth = Drive_Gear_Teeth / 3"
equation "Idle_Gear_Teeth = 10"
equation "Gear_Module = 2"
equation "Drive_Gear_Dia = ( Drive_Gear_Teeth * Gear_Module ) * 1 mm"
equation "Driven_Gear_Dia = ( Driven_Gear_Teeth * Gear_Module ) * 1 mm"
equation "Idle_Gear_Dia = ( Idle_Gear_Teeth * Gear_Module ) * 1 mm"
equation "Mount_Bolts = 8 mm"
equation "Mount_Bolt_Flange = 12 mm"
equation "Idle_Gear_Shaft = 8 mm"
equation "Gear_Clearance_Dia = 8 mm"
equation "d12 = Drive_Gear_Dia"
equation "d13 = Driven_Gear_Dia"
equation "d14 = Idle_Gear_Dia"
equation "d15 = Idle_Gear_Dia"
equation "d16 = Idle_Gear_Dia"
equation "Gear_Clearance_Drive = Gear_Clearance_Dia"
equation "d18 = Gear_Clearance_Dia"
equation "d19 = Mount_Bolt_Flange"
equation "d22 = Mount_Bolts"
equation "d23 = Gear_Clearance_Dia * 2.5"
equation "d24 = Idle_Gear_Shaft"
equation "d25 = Drive_Gear_Dia + Gear_Clearance_Dia"
equation "Drive_Gear_Shaft = 10 mm"
equation "Idle_Gear_Thickness = 21 mm"
equation "Gear_Thickness = 8 mm"
equation "Housing_Wall_Thickness = 3 mm"
equation "Gear_Gap = 5 mm"
equation "d32 = Gear_Thickness + Housing_Wall_Thickness"
equation "d33 = -Gear_Gap"
equation "d34 = -Gear_Gap - Gear_Thickness"
equation "d42 = Housing_Wall_Thickness"
equation "d44 = -Housing_Wall_Thickness - 1 mm"
equation "d50 = Housing_Wall_Thickness"
equation "d51 = d50"
equation "d55 = Gear_Clearance_Dia / 2"
equation "d57 = Gear_Clearance_Dia / 2"
equation "d58 = Gear_Thickness"
equation "d62 = Housing_Wall_Thickness - 1 mm"
equation "d66 = Housing_Wall_Thickness"
equation "d69 = -Housing_Wall_Thickness + 1 mm"
equation "d82 = Mount_Bolt_Flange"
equation "d95 = Mount_Bolt_Flange"
equation "d109 = Mount_Bolt_Flange"
equation "d110 = Mount_Bolt_Flange"
equation "d111 = Mount_Bolt_Flange"
named bodies: "Back Housing", "Front Housing", "Front Cover"
